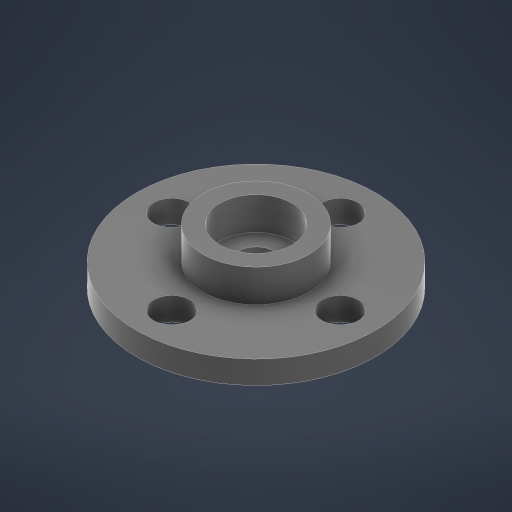
# Autodesk Inventor part: ServoDrive
Saved by Autodesk Inventor 2023 (Build 270158000, 158)
## iProperties
Created: 2023-02-24
Part Number: ServoDrive
Material: Steel
Document SubType Name: Modeling
Designer: roota
Density: 7.85 g/cm^3
Appearance: Smooth - Black
Mass: 265.715 g
Surface Area: 78.4173 cm^2
Volume: 33.849 cm^3
Author: roota
Autodesk Inventor part; units mm, degrees
ref_plane "YZ Plane" through (0, 0, 0) normal (1, 0, 0) x (0, 1, 0)
ref_plane "XZ Plane" through (0, 0, 0) normal (0, 1, 0) x (-1, 0, 0)
ref_plane "XY Plane" through (0, 0, 0) normal (0, 0, 1) x (1, 0, 0)
sketch "Sketch14" plane through (0, 0, 0) normal (0, 1, 0) x (-1, 0, 0)
  circle A0 centre (0, 0) radius 9.925
  circle A1 centre (0, 0) radius 7 construction
  circle A2 centre (7, 0) radius 1.5
  circle A3 centre (0, 7) radius 1.5
  circle A4 centre (-7, 0) radius 1.5
  circle A5 centre (0, -7) radius 1.5
  circle A6 centre (0, 0) radius 1.5
  dimension "d70" = 14
  dimension "d63" = 19.85
  dimension "d64" = 3
  dimension "d67" = 360
  dimension "d71" = 3
  constraints: 6 centre point, 3 coincident, 2 horizontal alignment, 11 other
  measures "d63" diameter of A0
  measures "d64" diameter of A2
  measures "d71" diameter of A6
extrude "Extrusion11" add sketch "Sketch14" along normal blind 1.9
sketch "Sketch15" plane through (0, 1.9, 0) normal (0, 1, 0) x (1, 0, 0)
  circle A0 centre (0, 0) radius 1.5 projected
  circle A1 centre (0, 0) radius 4.39
  circle A2 centre (0, 0) radius 3
  dimension "d74" = 8.78
  dimension "d75" = 6
  constraints: 2 centre point, 2 coincident
  measures "d74" diameter of A1
  measures "d75" diameter of A2
extrude "Extrusion12" add sketch "Sketch15" along normal blind 2.7 contours A1
body "Solid2"
